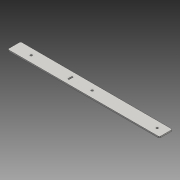
# Autodesk Inventor part: extension2
Saved by Autodesk Inventor 2016 (Build 200138000, 138)
## iProperties
Created: 2019-01-31
Part Number: extension2
Material: Generic
Document SubType Name: Modeling
Designer: TYP
Density: 1 g/cm^3
Appearance: Default
Author: TYP
Autodesk Inventor part; units mm, degrees
ref_plane "YZ Plane" through (0, 0, 0) normal (1, 0, 0) x (0, 1, 0)
ref_plane "XZ Plane" through (0, 0, 0) normal (0, 1, 0) x (-1, 0, 0)
ref_plane "XY Plane" through (0, 0, 0) normal (0, 0, 1) x (1, 0, 0)
sketch "Sketch1" plane through (0, 0, 0) normal (0, 0, 1) x (1, 0, 0)
  line L0 (-175, -15) -> (175, -15)
  line L1 (175, -15) -> (175, 15)
  line L2 (175, 15) -> (-175, 15)
  line L3 (-175, 15) -> (-175, -15)
  line L4 (-175, -15) -> (175, 15) construction
  line L5 (175, -15) -> (-175, 15) construction
  line L6 (-175, 0) -> (175, 0) construction
  circle A0 centre (155, 0) radius 2.25
  circle A1 centre (5, 0) radius 2.25
  circle A2 centre (-135.5, 0) radius 2.25
  point P0 (0, 0)
  dimension "d0" = 350
  dimension "d1" = 30
  dimension "d5" = 20
  dimension "d6" = 150
  dimension "d7" = 310.5
  dimension "d10" = 4.5
  dimension "d11" = 4.5
  dimension "d12" = 4.5
  constraints: 14 end point, 4 midpoint, 3 centre point, 3 point on line, 2 parallel, 1 horizontal, 1 perpendicular
  measures "d0" distance of L2.end L1.end
  measures "d1" distance of L1.end L0.end
  measures "d5" distance from line of L1 A0.centre
  measures "d6" distance of A1.centre A0.centre
  measures "d7" distance from line of A2.centre L1
  measures "d10" diameter of A1
  measures "d11" diameter of A0
  measures "d12" diameter of A2
extrude "Extrusion1" add sketch "Sketch1" along normal blind 3
sketch "Sketch2" plane through (0, 0, 3) normal (0, 0, 1) x (1, 0, 0)
  line L0 (-46.5, -5) -> (-43.5, -5)
  line L1 (-43.5, -5) -> (-43.5, 5)
  line L2 (-43.5, 5) -> (-46.5, 5)
  line L3 (-46.5, 5) -> (-46.5, -5)
  line L4 (-46.5, -5) -> (-43.5, 5) construction
  line L5 (-43.5, -5) -> (-46.5, 5) construction
  line L6 (175, -15) -> (175, 15) projected
  point P0 (0, 0)
  point P1 (-45, 0)
  point P2 (-45, 0)
  dimension "d13" = 3
  dimension "d14" = 10
  dimension "d15" = 220
  constraints: 12 end point, 3 midpoint, 2 parallel, 1 horizontal, 1 horizontal alignment, 1 perpendicular
  measures "d13" distance of L2.end L1.end
  measures "d14" distance of L1.end L0.end
  measures "d15" distance from line of L6 point (-45, 0)
extrude "Extrusion2" cut sketch "Sketch2" against normal through all
fillet "Fillet1" radius 3 4 edges at (-175, 15, 1.5) (-175, -15, 1.5) (175, -15, 1.5) (175, 15, 1.5)
equation "\"d16\" = d15"
body "Solid1"
